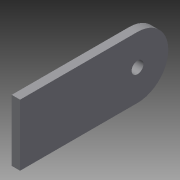
# Autodesk Inventor part: Suporte Motor
Saved by Autodesk Inventor 2015 (Build 190159000, 159)
## iProperties
Created: 2016-06-05
Part Number: Suporte Motor
Material: Generic
Document SubType Name: Modeling
Designer: EriveltonDell
Density: 1 g/cm^3
Appearance: Default
Author: EriveltonDell
Autodesk Inventor part; units mm, degrees
ref_plane "YZ Plane" through (0, 0, 0) normal (1, 0, 0) x (0, 1, 0)
ref_plane "XZ Plane" through (0, 0, 0) normal (0, 1, 0) x (-1, 0, 0)
ref_plane "XY Plane" through (0, 0, 0) normal (0, 0, 1) x (1, 0, 0)
sketch "Sketch3" plane through (0, 0, 0) normal (1, 0, 0) x (0, 1, 0)
  line L0 (0, 57) -> (0, 13)
  circle A0 centre (84, 35) radius 4.25
  line L1 (84, 35) -> (56.36, 35)
  line L2 (96, 53.4391) -> (92.6159, 55.2427)
  arc A1 (94.3473, 15.5852) -> (92.6159, 55.2427) centre (84, 35) ccw
  line L3 (84, 35) -> (71.3, 35)
  arc A2 (84, 13) -> (84, 57) centre (84, 35) ccw
  line L4 (84, 35) -> (84, 57)
  line L5 (0, 57) -> (84, 57)
  line L6 (84, 13) -> (0, 13)
  point P0 (0, 0)
  point P1 (84, 10.0705)
  point P2 (74.9172, 64.6754)
  dimension "d31" = 8.5
  dimension "d33" = 27.64
  dimension "d35" = 12.7
  dimension "d41" = 84
  constraints: 14 end point, 5 point on circle, 4 point on line, 3 centre point, 2 coincident, 2 perpendicular, 2 tangent, 1 concentric, 1 horizontal, 1 vertical
  measures "d31" diameter of A0
  measures "d33" distance of L1.start L1.end
  measures "d35" distance of L1.start L3.end
  measures "d41" distance from line of L0 A0.centre
extrude "Extrusion3" add sketch "Sketch3" along normal blind 6
body "Solid2"
